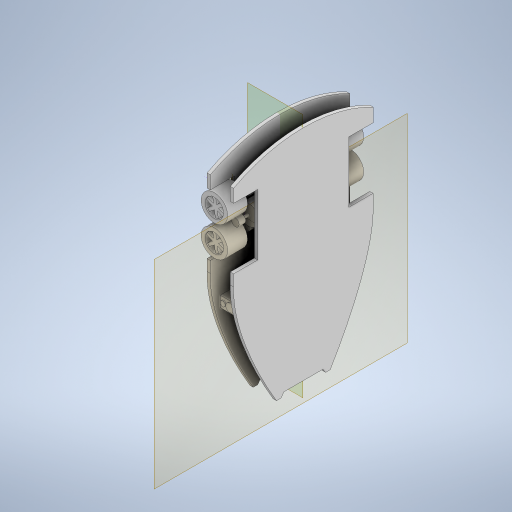
# Autodesk Inventor part: Mickey
Saved by Autodesk Inventor 2024 (Build 280153000, 153)
## iProperties
Created: 2024-01-30
Part Number: Mickey
Material: Generic
Document SubType Name: Modeling
Designer: Hitesh
Density: 1 g/cm^3
Appearance: Default
Author: Hitesh
Autodesk Inventor part; units mm, degrees
ref_plane "YZ Plane" through (0, 0, 0) normal (1, 0, 0) x (0, 1, 0)
ref_plane "XZ Plane" through (0, 0, 0) normal (0, 1, 0) x (-1, 0, 0)
ref_plane "XY Plane" through (0, 0, 0) normal (0, 0, 1) x (1, 0, 0)
sketch "Sketch1" plane through (0, 0, 0) normal (1, 0, 0) x (0, 1, 0)
  line L0 (79.528373, 42.408531) -> (71.671582, 42.408531)
  line L1 (34.839879, 42.408531) -> (28.023668, 42.408531)
  spline S0 degree 3 poles (28.023668, 42.408531) (8.43226, 43.15614) (-20.679837, 30.735066) (-44.361404, 16.548455) knots 0 0 0 0 1 1 1 1
  line L2 (-44.361404, 16.548455) -> (-44.361404, 13.844569)
  line L3 (-44.361404, 13.844569) -> (-41.928778, 12.127215)
  line L4 (-41.928778, 12.127215) -> (-41.928778, 0.037036)
  arc A0 (79.913681, -41.677922) -> (79.528373, 42.408531) centre (0, 0) ccw
  line L5 (79.913681, -41.677922) -> (71.671582, -41.677922)
  line L6 (34.839879, -41.677922) -> (28.023668, -41.677922)
  spline S1 degree 3 poles (28.023668, -41.677922) (8.431166, -42.471764) (-20.687268, -30.025765) (-44.361404, -15.817846) knots 0 0 0 0 1 1 1 1
  line L7 (-44.361404, -15.817846) -> (-44.361404, -13.113961)
  line L8 (-44.361404, -13.113961) -> (-41.928778, -11.396606)
  line L9 (-41.928778, -11.396606) -> (-41.928778, 0.037036)
  line L10 (34.839879, 42.408531) -> (34.839879, 27.893994)
  line L11 (34.839879, 27.893994) -> (71.671582, 27.893994)
  line L12 (71.671582, 27.893994) -> (71.671582, 42.408531)
  line L13 (34.839879, -41.677922) -> (34.839879, -27.163385)
  line L14 (34.839879, -27.163385) -> (71.671582, -27.163385)
  line L15 (71.671582, -27.163385) -> (71.671582, -41.677922)
  point P0 (9.125075, 40.060022)
  point P1 (-16.837429, 30.888781)
  point P2 (9.126574, -39.354229)
  point P3 (-16.837278, -30.181039)
  constraints: 32 end point, 2 parallel, 2 point on circle, 2 point on line, 2 vertical, 1 centre point, 1 coincident, 1 horizontal, 8 other
extrude "Extrusion1" add sketch "Sketch1" along normal blind 2
sketch "Sketch2" plane through (2, 0, 0) normal (1, 0, 0) x (0, 0, -1)
  line L0 (-42.408531, 71.671582) -> (-27.893994, 71.671582) construction
  line L1 (-27.893994, 34.839879) -> (-42.408531, 34.839879) construction
  line L2 (-42.408531, 71.671582) -> (-42.408531, 34.839879) construction
  line L3 (-42.408531, 53.25573) -> (49.70936, 53.25573) construction
  line L4 (-27.893994, 71.671582) -> (-27.893994, 34.839879) construction
  line L5 (41.677922, 34.839879) -> (27.163385, 34.839879) construction
  line L6 (-11.47496, 42.729901) -> (11.47496, 42.729901) construction
  line L7 (11.47496, 42.729901) -> (11.47496, 26.949856) construction
  line L8 (11.47496, 26.949856) -> (-11.47496, 26.949856) construction
  line L9 (-11.47496, 26.949856) -> (-11.47496, 42.729901) construction
  line L10 (-11.47496, 42.729901) -> (11.47496, 26.949856) construction
  line L11 (11.47496, 42.729901) -> (-11.47496, 26.949856) construction
  line L12 (-11.47496, 34.839879) -> (11.47496, 34.839879)
  line L13 (11.47496, 34.839879) -> (11.47496, 19.846275)
  line L14 (11.47496, 19.846275) -> (-11.47496, 19.846275)
  line L15 (-11.47496, 19.846275) -> (-11.47496, 34.839879)
  line L16 (-7.0791, 16.000261) -> (7.117483, 16.000261)
  line L17 (7.117483, 16.000261) -> (7.117483, 4.324761)
  line L18 (7.117483, 4.324761) -> (-7.0791, 4.324761)
  line L19 (-7.0791, 4.324761) -> (-7.0791, 16.000261)
  point P0 (0, 0)
  point P1 (0, 34.839879)
  constraints: 32 end point, 6 parallel, 4 horizontal, 4 midpoint, 3 perpendicular, 1 vertical
extrude "Extrusion2" add sketch "Sketch2" along normal blind 2
sketch "Sketch3" plane through (2, 0, 0) normal (1, 0, 0) x (0, 0, -1)
  line L0 (7.117483, 16.000261) -> (-7.0791, 16.000261) construction
  line L1 (7.117483, 16.000261) -> (7.117483, 4.324761) construction
  line L2 (-7.0791, 16.000261) -> (7.117483, 16.000261) construction
  line L3 (7.117483, 16.000261) -> (7.117483, 4.324761) construction
  line L4 (7.117483, 4.324761) -> (-7.0791, 4.324761) construction
  line L5 (-7.0791, 4.324761) -> (-7.0791, 16.000261) construction
  line L6 (-6.840727, 16.000261) -> (-6.494492, 16.000261)
  line L7 (-6.494492, 16.000261) -> (-6.494492, 17.001112)
  line L8 (-6.494492, 17.001112) -> (-6.840727, 17.001112)
  line L9 (-6.840727, 17.001112) -> (-6.840727, 16.000261)
  line L10 (-5.820727, 16.000261) -> (-5.474492, 16.000261)
  line L11 (-5.474492, 16.000261) -> (-5.474492, 17.001112)
  line L12 (-5.474492, 17.001112) -> (-5.820727, 17.001112)
  line L13 (-5.820727, 17.001112) -> (-5.820727, 16.000261)
  line L14 (-4.800727, 16.000261) -> (-4.454492, 16.000261)
  line L15 (-4.454492, 16.000261) -> (-4.454492, 17.001112)
  line L16 (-4.454492, 17.001112) -> (-4.800727, 17.001112)
  line L17 (-4.800727, 17.001112) -> (-4.800727, 16.000261)
  line L18 (-3.780727, 16.000261) -> (-3.434492, 16.000261)
  line L19 (-3.434492, 16.000261) -> (-3.434492, 17.001112)
  line L20 (-3.434492, 17.001112) -> (-3.780727, 17.001112)
  line L21 (-3.780727, 17.001112) -> (-3.780727, 16.000261)
  line L22 (-2.760727, 16.000261) -> (-2.414492, 16.000261)
  line L23 (-2.414492, 16.000261) -> (-2.414492, 17.001112)
  line L24 (-2.414492, 17.001112) -> (-2.760727, 17.001112)
  line L25 (-2.760727, 17.001112) -> (-2.760727, 16.000261)
  line L26 (-1.740727, 16.000261) -> (-1.394492, 16.000261)
  line L27 (-1.394492, 16.000261) -> (-1.394492, 17.001112)
  line L28 (-1.394492, 17.001112) -> (-1.740727, 17.001112)
  line L29 (-1.740727, 17.001112) -> (-1.740727, 16.000261)
  line L30 (-0.720727, 16.000261) -> (-0.374492, 16.000261)
  line L31 (-0.374492, 16.000261) -> (-0.374492, 17.001112)
  line L32 (-0.374492, 17.001112) -> (-0.720727, 17.001112)
  line L33 (-0.720727, 17.001112) -> (-0.720727, 16.000261)
  line L34 (0.299273, 16.000261) -> (0.645508, 16.000261)
  line L35 (0.645508, 16.000261) -> (0.645508, 17.001112)
  line L36 (0.645508, 17.001112) -> (0.299273, 17.001112)
  line L37 (0.299273, 17.001112) -> (0.299273, 16.000261)
  line L38 (1.319273, 16.000261) -> (1.665508, 16.000261)
  line L39 (1.665508, 16.000261) -> (1.665508, 17.001112)
  line L40 (1.665508, 17.001112) -> (1.319273, 17.001112)
  line L41 (1.319273, 17.001112) -> (1.319273, 16.000261)
  line L42 (2.339273, 16.000261) -> (2.685508, 16.000261)
  line L43 (2.685508, 16.000261) -> (2.685508, 17.001112)
  line L44 (2.685508, 17.001112) -> (2.339273, 17.001112)
  line L45 (2.339273, 17.001112) -> (2.339273, 16.000261)
  line L46 (3.359273, 16.000261) -> (3.705508, 16.000261)
  line L47 (3.705508, 16.000261) -> (3.705508, 17.001112)
  line L48 (3.705508, 17.001112) -> (3.359273, 17.001112)
  line L49 (3.359273, 17.001112) -> (3.359273, 16.000261)
  line L50 (4.379273, 16.000261) -> (4.725508, 16.000261)
  line L51 (4.725508, 16.000261) -> (4.725508, 17.001112)
  line L52 (4.725508, 17.001112) -> (4.379273, 17.001112)
  line L53 (4.379273, 17.001112) -> (4.379273, 16.000261)
  line L54 (5.399273, 16.000261) -> (5.745508, 16.000261)
  line L55 (5.745508, 16.000261) -> (5.745508, 17.001112)
  line L56 (5.745508, 17.001112) -> (5.399273, 17.001112)
  line L57 (5.399273, 17.001112) -> (5.399273, 16.000261)
  line L58 (6.419273, 16.000261) -> (6.765508, 16.000261)
  line L59 (6.765508, 16.000261) -> (6.765508, 17.001112)
  line L60 (6.765508, 17.001112) -> (6.419273, 17.001112)
  line L61 (6.419273, 17.001112) -> (6.419273, 16.000261)
  line L62 (-7.0791, 10.162511) -> (7.117483, 10.162511) construction
  circle A0 centre (0.019192, 10.162511) radius 1.15053 construction
  line L63 (3.81911, 3.323909) -> (3.81911, 4.324761)
  line L64 (3.81911, 4.324761) -> (3.472876, 4.324761)
  line L65 (3.472876, 3.323909) -> (3.81911, 3.323909)
  line L66 (3.472876, 4.324761) -> (3.472876, 3.323909)
  line L67 (2.79911, 3.323909) -> (2.79911, 4.324761)
  line L68 (2.79911, 4.324761) -> (2.452876, 4.324761)
  line L69 (2.452876, 4.324761) -> (2.452876, 3.323909)
  line L70 (1.77911, 3.323909) -> (1.77911, 4.324761)
  line L71 (1.77911, 4.324761) -> (1.432876, 4.324761)
  line L72 (1.432876, 4.324761) -> (1.432876, 3.323909)
  line L73 (1.432876, 3.323909) -> (1.77911, 3.323909)
  line L74 (2.452876, 3.323909) -> (2.79911, 3.323909)
  line L75 (0.75911, 3.323909) -> (0.75911, 4.324761)
  line L76 (0.412876, 3.323909) -> (0.75911, 3.323909)
  line L77 (0.75911, 4.324761) -> (0.412876, 4.324761)
  line L78 (0.412876, 4.324761) -> (0.412876, 3.323909)
  line L79 (-0.26089, 3.323909) -> (-0.26089, 4.324761)
  line L80 (-0.26089, 4.324761) -> (-0.607124, 4.324761)
  line L81 (-0.607124, 3.323909) -> (-0.26089, 3.323909)
  line L82 (-1.28089, 3.323909) -> (-1.28089, 4.324761)
  line L83 (-1.627124, 4.324761) -> (-1.627124, 3.323909)
  line L84 (-1.28089, 4.324761) -> (-1.627124, 4.324761)
  line L85 (-1.627124, 3.323909) -> (-1.28089, 3.323909)
  line L86 (-0.607124, 4.324761) -> (-0.607124, 3.323909)
  line L87 (-2.30089, 3.323909) -> (-2.30089, 4.324761)
  line L88 (-2.647124, 3.323909) -> (-2.30089, 3.323909)
  line L89 (-2.30089, 4.324761) -> (-2.647124, 4.324761)
  line L90 (-2.647124, 4.324761) -> (-2.647124, 3.323909)
  line L91 (-3.32089, 3.323909) -> (-3.32089, 4.324761)
  line L92 (-3.32089, 4.324761) -> (-3.667124, 4.324761)
  line L93 (-3.667124, 3.323909) -> (-3.32089, 3.323909)
  line L94 (-4.34089, 3.323909) -> (-4.34089, 4.324761)
  line L95 (-4.34089, 4.324761) -> (-4.687124, 4.324761)
  line L96 (-4.687124, 3.323909) -> (-4.34089, 3.323909)
  line L97 (-5.36089, 3.323909) -> (-5.36089, 4.324761)
  line L98 (-5.36089, 4.324761) -> (-5.707124, 4.324761)
  line L99 (-5.707124, 3.323909) -> (-5.36089, 3.323909)
  line L100 (-6.38089, 3.323909) -> (-6.38089, 4.324761)
  line L101 (-6.38089, 4.324761) -> (-6.727124, 4.324761)
  line L102 (-6.727124, 4.324761) -> (-6.727124, 3.323909)
  line L103 (-6.727124, 3.323909) -> (-6.38089, 3.323909)
  line L104 (-3.667124, 4.324761) -> (-3.667124, 3.323909)
  line L105 (6.87911, 4.324761) -> (6.532876, 4.324761)
  line L106 (6.532876, 4.324761) -> (6.532876, 3.323909)
  line L107 (6.532876, 3.323909) -> (6.87911, 3.323909)
  line L108 (6.87911, 3.323909) -> (6.87911, 4.324761)
  line L109 (5.85911, 4.324761) -> (5.512876, 4.324761)
  line L110 (5.512876, 4.324761) -> (5.512876, 3.323909)
  line L111 (5.512876, 3.323909) -> (5.85911, 3.323909)
  line L112 (4.492876, 4.324761) -> (4.492876, 3.323909)
  line L113 (4.83911, 4.324761) -> (4.492876, 4.324761)
  line L114 (4.83911, 3.323909) -> (4.83911, 4.324761)
  line L115 (5.85911, 3.323909) -> (5.85911, 4.324761)
  line L116 (4.492876, 3.323909) -> (4.83911, 3.323909)
  line L117 (-4.687124, 4.324761) -> (-4.687124, 3.323909)
  line L118 (-5.707124, 4.324761) -> (-5.707124, 3.323909)
  line L119 (7.117483, 4.324761) -> (-7.0791, 4.324761) construction
  line L120 (8.115724, 15.294592) -> (8.115724, 15.640827)
  line L121 (8.115724, 15.640827) -> (7.117483, 15.640827)
  line L122 (7.117483, 15.640827) -> (7.117483, 15.294592)
  line L123 (7.117483, 15.294592) -> (8.115724, 15.294592)
  line L124 (7.117483, 4.324761) -> (7.117483, 16.000261) construction
  line L125 (7.117483, 14.610827) -> (7.117483, 14.264592)
  line L126 (8.115724, 14.610827) -> (7.117483, 14.610827)
  line L127 (8.115724, 14.264592) -> (8.115724, 14.610827)
  line L128 (7.117483, 14.264592) -> (8.115724, 14.264592)
  line L129 (7.117483, 13.580827) -> (7.117483, 13.234592)
  line L130 (8.115724, 13.580827) -> (7.117483, 13.580827)
  line L131 (8.115724, 13.234592) -> (8.115724, 13.580827)
  line L132 (7.117483, 13.234592) -> (8.115724, 13.234592)
  line L133 (7.117483, 12.550827) -> (7.117483, 12.204592)
  line L134 (8.115724, 12.550827) -> (7.117483, 12.550827)
  line L135 (8.115724, 12.204592) -> (8.115724, 12.550827)
  line L136 (7.117483, 12.204592) -> (8.115724, 12.204592)
  line L137 (7.117483, 11.520827) -> (7.117483, 11.174592)
  line L138 (8.115724, 11.520827) -> (7.117483, 11.520827)
  line L139 (8.115724, 11.174592) -> (8.115724, 11.520827)
  line L140 (7.117483, 11.174592) -> (8.115724, 11.174592)
  line L141 (7.117483, 10.490827) -> (7.117483, 10.144592)
  line L142 (8.115724, 10.490827) -> (7.117483, 10.490827)
  line L143 (8.115724, 10.144592) -> (8.115724, 10.490827)
  line L144 (7.117483, 10.144592) -> (8.115724, 10.144592)
  line L145 (7.117483, 9.460827) -> (7.117483, 9.114592)
  line L146 (8.115724, 9.460827) -> (7.117483, 9.460827)
  line L147 (8.115724, 9.114592) -> (8.115724, 9.460827)
  line L148 (7.117483, 9.114592) -> (8.115724, 9.114592)
  line L149 (7.117483, 8.430827) -> (7.117483, 8.084592)
  line L150 (8.115724, 8.430827) -> (7.117483, 8.430827)
  line L151 (8.115724, 8.084592) -> (8.115724, 8.430827)
  line L152 (7.117483, 8.084592) -> (8.115724, 8.084592)
  line L153 (7.117483, 7.400827) -> (7.117483, 7.054592)
  line L154 (8.115724, 7.400827) -> (7.117483, 7.400827)
  line L155 (8.115724, 7.054592) -> (8.115724, 7.400827)
  line L156 (7.117483, 7.054592) -> (8.115724, 7.054592)
  line L157 (7.117483, 6.370827) -> (7.117483, 6.024592)
  line L158 (8.115724, 6.370827) -> (7.117483, 6.370827)
  line L159 (8.115724, 6.024592) -> (8.115724, 6.370827)
  line L160 (7.117483, 6.024592) -> (8.115724, 6.024592)
  line L161 (7.117483, 5.340827) -> (7.117483, 4.994592)
  line L162 (8.115724, 5.340827) -> (7.117483, 5.340827)
  line L163 (8.115724, 4.994592) -> (8.115724, 5.340827)
  line L164 (7.117483, 4.994592) -> (8.115724, 4.994592)
  line L165 (0.019192, 12.377709) -> (0.019192, 7.657773) construction
  line L166 (-7.0791, 16.000261) -> (-7.0791, 4.324761) construction
  line L167 (-7.0791, 16.000261) -> (-7.0791, 4.324761) construction
  line L168 (-7.0791, 15.294592) -> (-8.077341, 15.294592)
  line L169 (-7.0791, 15.640827) -> (-7.0791, 15.294592)
  line L170 (-8.077341, 15.640827) -> (-7.0791, 15.640827)
  line L171 (-8.077341, 15.294592) -> (-8.077341, 15.640827)
  line L172 (-7.0791, 4.324761) -> (-7.0791, 16.000261) construction
  line L173 (-7.0791, 14.610827) -> (-7.0791, 14.264592)
  line L174 (-8.077341, 14.610827) -> (-7.0791, 14.610827)
  line L175 (-8.077341, 14.264592) -> (-8.077341, 14.610827)
  line L176 (-7.0791, 14.264592) -> (-8.077341, 14.264592)
  line L177 (-7.0791, 13.580827) -> (-7.0791, 13.234592)
  line L178 (-8.077341, 13.580827) -> (-7.0791, 13.580827)
  line L179 (-8.077341, 13.234592) -> (-8.077341, 13.580827)
  line L180 (-7.0791, 13.234592) -> (-8.077341, 13.234592)
  line L181 (-7.0791, 12.550827) -> (-7.0791, 12.204592)
  line L182 (-8.077341, 12.550827) -> (-7.0791, 12.550827)
  line L183 (-8.077341, 12.204592) -> (-8.077341, 12.550827)
  line L184 (-7.0791, 12.204592) -> (-8.077341, 12.204592)
  line L185 (-7.0791, 11.520827) -> (-7.0791, 11.174592)
  line L186 (-8.077341, 11.520827) -> (-7.0791, 11.520827)
  line L187 (-8.077341, 11.174592) -> (-8.077341, 11.520827)
  line L188 (-7.0791, 11.174592) -> (-8.077341, 11.174592)
  line L189 (-7.0791, 10.490827) -> (-7.0791, 10.144592)
  line L190 (-8.077341, 10.490827) -> (-7.0791, 10.490827)
  line L191 (-8.077341, 10.144592) -> (-8.077341, 10.490827)
  line L192 (-7.0791, 10.144592) -> (-8.077341, 10.144592)
  line L193 (-7.0791, 9.460827) -> (-7.0791, 9.114592)
  line L194 (-8.077341, 9.460827) -> (-7.0791, 9.460827)
  line L195 (-8.077341, 9.114592) -> (-8.077341, 9.460827)
  line L196 (-7.0791, 9.114592) -> (-8.077341, 9.114592)
  line L197 (-7.0791, 8.430827) -> (-7.0791, 8.084592)
  line L198 (-8.077341, 8.430827) -> (-7.0791, 8.430827)
  line L199 (-8.077341, 8.084592) -> (-8.077341, 8.430827)
  line L200 (-7.0791, 8.084592) -> (-8.077341, 8.084592)
  line L201 (-7.0791, 7.400827) -> (-7.0791, 7.054592)
  line L202 (-8.077341, 7.400827) -> (-7.0791, 7.400827)
  line L203 (-8.077341, 7.054592) -> (-8.077341, 7.400827)
  line L204 (-7.0791, 7.054592) -> (-8.077341, 7.054592)
  line L205 (-7.0791, 6.370827) -> (-7.0791, 6.024592)
  line L206 (-8.077341, 6.370827) -> (-7.0791, 6.370827)
  line L207 (-8.077341, 6.024592) -> (-8.077341, 6.370827)
  line L208 (-7.0791, 6.024592) -> (-8.077341, 6.024592)
  line L209 (-7.0791, 5.340827) -> (-7.0791, 4.994592)
  line L210 (-8.077341, 5.340827) -> (-7.0791, 5.340827)
  line L211 (-8.077341, 4.994592) -> (-8.077341, 5.340827)
  line L212 (-7.0791, 4.994592) -> (-8.077341, 4.994592)
  point P0 (0, 0)
  dimension "d21" = 1.02
  dimension "d28" = 360
  dimension "d32" = 1.03
  constraints: 420 end point, 48 symmetric about line, 4 parallel, 3 horizontal, 3 midpoint, 2 perpendicular, 2 point on line, 2 vertical, 1 centre point, 1 collinear, 415 other
  measures "d21" distance of L6.start L10.start
  measures "d32" distance of L123.start L125.end
extrude "Extrusion3" add sketch "Sketch3" along normal blind 1.5
sketch "Sketch4" plane through (2, 4.994592, -8.115724) normal (0, -1, 0) x (1, 0, 0)
  line L0 (1.5, 0.998241) -> (0, 0.998241)
  line L1 (0, 0.998241) -> (1, 0.998241)
  line L2 (1, 0.998241) -> (1, 0.498241)
  line L3 (1, 0.498241) -> (0, 0.498241)
  line L4 (0, 0.498241) -> (0, 0.998241)
  line L5 (0, 15.694824) -> (1, 15.694824)
  line L6 (1, 15.694824) -> (1, 15.194824)
  line L7 (1, 15.194824) -> (0, 15.194824)
  line L8 (0, 15.194824) -> (0, 15.694824)
  line L9 (0, 15.194824) -> (2, 15.194824)
  line L10 (0, 20.242939) -> (0, -3.280882)
  point P0 (-2, 8.115724)
  point P1 (1, 0.998241)
  dimension "d39" = 1
  dimension "d40" = 0.5
  dimension "d41" = 1
  dimension "d42" = 0.5
  constraints: 16 end point, 4 parallel, 2 collinear, 2 horizontal, 2 perpendicular
  measures "d39" distance of L2.end L3.end
  measures "d40" distance of L1.end L2.end
  measures "d41" distance of L6.end L7.end
  measures "d42" distance of L5.end L6.end
extrude "Extrusion4" cut sketch "Sketch4" against normal up to surface (14.851683 mm away)
sketch "Sketch5" plane through (2, 16.000261, 6.840727) normal (0, 0, 1) x (1, 0, 0)
  line L0 (0, -11.6755) -> (1, -11.6755)
  line L1 (1, -11.6755) -> (1, -12.1755)
  line L2 (1, -12.1755) -> (0, -12.1755)
  line L3 (0, -12.1755) -> (0, -11.6755)
  line L4 (0, -11.6755) -> (2, -11.6755)
  line L5 (0, -12.676351) -> (0, -11.6755)
  line L6 (0, 0.5) -> (1, 0.5)
  line L7 (1, 0.5) -> (1, 0)
  line L8 (1, 0) -> (0, 0)
  line L9 (0, 0) -> (0, 0.5)
  line L10 (0, 0) -> (2, 0)
  line L11 (0, 0) -> (0, 1.000851)
  point P0 (-2, -16.000261)
  dimension "d45" = 1
  dimension "d46" = 0.5
  dimension "d47" = 1
  dimension "d48" = 0.5
  constraints: 16 end point, 4 collinear, 4 parallel, 2 horizontal, 2 perpendicular
  measures "d45" distance of L1.end L2.end
  measures "d46" distance of L0.end L1.end
  measures "d47" distance of L7.end L8.end
  measures "d48" distance of L6.end L7.end
extrude "Extrusion5" cut sketch "Sketch5" against normal through all
sketch "Sketch6" plane through (0, 34.839879, 27.893994) normal (0, 0, 1) x (1, 0, 0)
  line L0 (0, 36.831703) -> (0, 0) construction
  line L1 (0, 18.415852) -> (14.226225, 18.415852) construction
  line L2 (8.271561, 36.831703) -> (8.271561, 18.415852) construction
  line L3 (8.271561, 27.623777) -> (-16.043318, 27.623777) construction
  line L4 (3.408585, 18.415852) -> (3.408585, 0) construction
  point P0 (0, -34.839879)
  constraints: 8 end point, 2 horizontal, 2 midpoint, 2 point on line, 1 perpendicular, 1 vertical
ref_plane "Work Plane1" through (0, 34.839879, 29.393994) normal (0, 0, 1) x (1, 0, 0)
sketch "Sketch7" plane through (0, 34.839879, 29.393994) normal (0, 0, 1) x (1, 0, 0)
  line L0 (3.388556, 18.455419) -> (3.388556, 36.831703) construction
  circle A0 centre (3.388556, 27.643561) radius 8
  line L1 (3.388556, 18.455419) -> (3.388556, 0.120115) construction
  circle A1 centre (3.388556, 9.287767) radius 8
  point P0 (0, -34.839879)
  dimension "d52" = 16
  dimension "d53" = 16
  constraints: 4 end point, 2 centre point, 2 midpoint, 2 vertical
  measures "d52" diameter of A0
  measures "d53" diameter of A1
extrude "Extrusion6" add sketch "Sketch7" along normal blind 12
sketch "Sketch8" plane through (3.388556, 62.48344, 29.393994) normal (0, 0, -1) x (-1, 0, 0)
  circle A0 centre (0, 0) radius 1.045344 construction
  circle A1 centre (0, 0) radius 0.75
  circle A2 centre (0, -18.355794) radius 8
  circle A3 centre (0, -18.355794) radius 0.75
  point P0 (3.388556, -62.48344)
  dimension "d56" = 1.5
  dimension "d57" = 1.5
  constraints: 3 centre point, 2 coincident
  measures "d56" diameter of A1
  measures "d57" diameter of A3
extrude "Extrusion7" add sketch "Sketch8" along normal blind 6 contours A1 | A3
sketch "Sketch9" plane through (3.388556, 62.48344, 23.393994) normal (0, 0, -1) x (-1, 0, 0)
  circle A0 centre (0, 0) radius 0.75
  arc A1 (1.388556, 2.659307) -> (1.388556, -2.659307) centre (0, 0) ccw
  line L0 (1.388556, 9.188142) -> (1.388556, -27.643561)
  line L1 (1.388556, 2.659307) -> (1.388556, -2.659307)
  circle A2 centre (0, -18.355794) radius 0.75
  arc A3 (1.388556, -15.696487) -> (1.388556, -21.015101) centre (0, -18.355794) ccw
  line L2 (1.388556, -15.696487) -> (1.388556, -21.015101)
  point P0 (3.388556, -62.48344)
  dimension "d60" = 3
  dimension "d61" = 6
  constraints: 4 end point, 4 point on circle, 4 point on line, 2 centre point, 2 coincident
  measures "d60" radius of A1
  measures "d61" diameter of A3
extrude "Extrusion8" add sketch "Sketch9" along normal blind 4 contours A0 | L0 A1 | L0 A3 | A2
sketch "Sketch10" plane through (3.388556, 62.48344, 23.393994) normal (0, 0, 1) x (1, 0, 0)
  line L0 (-1.388556, 9.188142) -> (-1.388556, -27.643561)
  circle A0 centre (4.628085, -9.227709) radius 6.016657
  point P0 (-3.388556, -62.48344)
  constraints: 1 centre point
extrude "Extrusion9" add sketch "Sketch10" along normal blind 2 and the other way blind 16
sketch "Sketch11" plane through (3.388556, 62.48344, 25.393994) normal (0, 0, 1) x (1, 0, 0)
  arc A0 (-1.388556, -9.241554) -> (-1.388556, -9.213864) centre (4.628085, -9.227709) ccw
  circle A1 centre (4.628085, -9.227709) radius 0.75
  point P0 (-3.388556, -62.48344)
  dimension "d69" = 1.5
  constraints: 1 centre point, 1 coincident
  measures "d69" diameter of A1
extrude "Extrusion10" add sketch "Sketch11" along normal blind 8
sketch "Sketch12" plane through (8.016641, 53.25573, 33.393994) normal (0, 0, 1) x (1, 0, 0)
  circle A0 centre (0, 0) radius 2.323265
  circle A1 centre (-4.628085, 9.227709) radius 8
  point P0 (-8.016641, -53.25573)
  constraints: 1 centre point, 1 tangent
extrude "Extrusion11" add sketch "Sketch12" against normal blind 4 contours A0
ref_plane "Work Plane2" through (0, 34.839879, 0.365304) normal (0, 0, -1) x (-1, 0, 0)
mirror "Mirror1" about plane through (0, 34.839879, 0.365304) normal (0, 0, -1) of "Extrusion6", "Extrusion11", "Extrusion10", "Extrusion9", "Extrusion8", "Extrusion7"
sketch "Sketch13" plane through (3.388556, 62.48344, 41.393994) normal (0, 0, 1) x (1, 0, 0)
  circle A0 centre (0, 0) radius 5.585986
  line L0 (-3.794465, -4.201608) -> (4.942451, 2.761097)
  line L1 (4.942451, 2.761097) -> (3.794465, 4.201608)
  line L2 (3.794465, 4.201608) -> (-4.942451, -2.761097)
  line L3 (-4.942451, -2.761097) -> (-3.794465, -4.201608)
  line L4 (-3.794465, -4.201608) -> (3.794465, 4.201608) construction
  line L5 (4.942451, 2.761097) -> (-4.942451, -2.761097) construction
  line L6 (1.741467, -5.386907) -> (0.080046, 5.660837)
  line L7 (-1.741467, 5.386907) -> (-0.080046, -5.660837)
  line L8 (5.535932, -1.185299) -> (-4.862405, 2.89974)
  line L9 (-5.535932, 1.185299) -> (4.862405, -2.89974)
  line L10 (3.794465, 4.201608) -> (-4.942451, -2.761097)
  line L11 (-3.794465, -4.201608) -> (4.942451, 2.761097)
  line L12 (-1.741467, 5.386907) -> (-0.080046, -5.660837)
  line L13 (1.741467, -5.386907) -> (0.080046, 5.660837)
  line L14 (-5.535932, 1.185299) -> (4.862405, -2.89974)
  line L15 (5.535932, -1.185299) -> (-4.862405, 2.89974)
  circle A1 centre (0, -18.330655) radius 5.585986
  line L16 (-3.794465, -22.532263) -> (4.942451, -15.569559)
  line L17 (4.942451, -15.569559) -> (3.794465, -14.129047)
  line L18 (3.794465, -14.129047) -> (-4.942451, -21.091752)
  line L19 (-4.942451, -21.091752) -> (-3.794465, -22.532263)
  line L20 (-3.794465, -22.532263) -> (3.794465, -14.129047) construction
  line L21 (4.942451, -15.569559) -> (-4.942451, -21.091752) construction
  line L22 (1.741467, -23.717562) -> (0.080046, -12.669819)
  line L23 (-1.741467, -12.943748) -> (-0.080046, -23.991492)
  line L24 (5.535932, -19.515954) -> (-4.862405, -15.430915)
  line L25 (-5.535932, -17.145356) -> (4.862405, -21.230395)
  line L26 (3.794465, -14.129047) -> (-4.942451, -21.091752)
  line L27 (-3.794465, -22.532263) -> (4.942451, -15.569559)
  line L28 (-1.741467, -12.943748) -> (-0.080046, -23.991492)
  line L29 (1.741467, -23.717562) -> (0.080046, -12.669819)
  line L30 (-5.535932, -17.145356) -> (4.862405, -21.230395)
  line L31 (5.535932, -19.515954) -> (-4.862405, -15.430915)
  point P0 (-3.388556, -62.48344)
  point P1 (-4.791251, 2.871787)
  point P2 (-1.147986, 1.440512)
  point P3 (-1.730098, 5.311309)
  point P4 (-1.821513, -0.273929)
  point P5 (-5.464777, 1.157346)
  point P6 (-4.882665, -2.713452)
  point P7 (-0.091415, -5.585238)
  point P8 (-0.673527, -1.714441)
  point P9 (-3.734679, -4.153963)
  point P10 (4.791251, -2.871787)
  point P11 (1.147986, -1.440512)
  point P12 (1.730098, -5.311309)
  point P13 (1.821513, 0.273929)
  point P14 (5.464777, -1.157346)
  point P15 (4.882665, 2.713452)
  point P16 (0.091415, 5.585238)
  point P17 (0.673527, 1.714441)
  point P18 (3.734679, 4.153963)
  point P19 (1.147986, -19.771167)
  point P20 (1.730098, -23.641964)
  point P21 (4.791251, -21.202442)
  point P22 (-0.091415, -23.915893)
  point P23 (-0.673527, -20.045096)
  point P24 (-3.734679, -22.484618)
  point P25 (-1.821513, -18.604584)
  point P26 (-5.464777, -17.17331)
  point P27 (-4.882665, -21.044107)
  point P28 (-1.147986, -16.890143)
  point P29 (-1.730098, -13.019346)
  point P30 (-4.791251, -15.458869)
  point P31 (0.091415, -12.745417)
  point P32 (0.673527, -16.616214)
  point P33 (3.734679, -14.176692)
  point P34 (1.821513, -18.056726)
  point P35 (5.464777, -19.488001)
  point P36 (4.882665, -15.617204)
  dimension "d76" = 360
  dimension "d84" = 360
  constraints: 64 end point, 4 midpoint, 4 parallel, 2 centre point, 2 perpendicular, 74 other
extrude "Extrusion12" cut sketch "Sketch13" against normal blind 6 contours A0 L8 L0 | A0 L6 L9 | L2 L6 A0 | A0 L0 L7 | L7 L8 A0 | L2 A0 L9 | A1 L24 L16 | A1 L22 L25 | L18 L22 A1 | A1 L16 L23 | L23 L24 A1 | L18 A1 L25
sketch "Sketch14" plane through (3.388556, 62.48344, 41.393994) normal (0, 0, 1) x (1, 0, 0)
  circle A0 centre (0, 0) radius 5.585986
  arc A1 (1.730098, -23.641964) -> (4.791251, -21.202442) centre (0, -18.330655) ccw
  circle A2 centre (0, -18.330655) radius 5.585986
  point P0 (-3.388556, -62.48344)
  constraints: 2 centre point, 1 coincident
extrude "Extrusion13" cut sketch "Sketch14" against normal blind 0.7
mirror "Mirror2" about plane through (0, 34.839879, 0.365304) normal (0, 0, -1) of "Extrusion13", "Extrusion12", "Extrusion6"
sketch "Sketch15" plane through (2, 0, 0) normal (1, 0, 0) x (0, 0, -1)
  line L0 (-13.844569, -44.361404) -> (-13.844569, 2.739873) construction
  line L1 (-13.844569, 2.739873) -> (13.113961, 2.739873) construction
  line L2 (13.113961, -44.361404) -> (15.817846, -44.361404) construction
  line L3 (13.113961, 2.739873) -> (13.113961, -44.361404) construction
  line L4 (-13.844569, -20.810765) -> (-17.838326, -25.941355)
  line L5 (-17.838326, -25.941355) -> (-22.283823, -22.480889)
  line L6 (-22.283823, -22.480889) -> (-18.290067, -17.350299)
  line L7 (-18.290067, -17.350299) -> (-13.844569, -20.810765)
  line L8 (-30.753552, 13.664836) -> (-30.764664, 7.163074)
  line L9 (-30.764664, 7.163074) -> (-36.39824, 7.172702)
  line L10 (-36.39824, 7.172702) -> (-36.387128, 13.674464)
  line L11 (-36.387128, 13.674464) -> (-30.753552, 13.664836)
  point P0 (0, 0)
  constraints: 22 end point, 4 parallel, 4 perpendicular, 1 midpoint, 1 vertical
extrude "Extrusion14" add sketch "Sketch15" along normal blind 9
sketch "Sketch16" plane through (2, -25.941355, 17.838326) normal (0, -0.7891064, 0.6142566) x (1, 0, 0)
  line L0 (0, 5.633584) -> (9, 5.633584) construction
  line L1 (0, 0) -> (9, 0) construction
  line L2 (0, 5.633584) -> (9, 0) construction
  line L3 (6.271221, -0.889158) -> (6.271221, 3.293106)
  circle A0 centre (6.271221, 2.816792) radius 2.517328
  circle A1 centre (1.994855, 2.816792) radius 1.587953
  point P0 (-2, 1.858311)
  constraints: 2 centre point, 2 end point, 1 point on line
extrude "Extrusion15" add sketch "Sketch16" along normal blind 0.5
sketch "Sketch17" plane through (2, 7.172702, 36.39824) normal (0, 0.001709, 0.9999985) x (1, 0, 0)
  circle A0 centre (6.240376, 3.24716) radius 2.517328
  circle A1 centre (1.964009, 3.24716) radius 1.587953
  line L0 (0, 6.501772) -> (9, 6.501772) construction
  line L1 (4.5, 6.501772) -> (4.5, 0) construction
  line L2 (0, 0) -> (9, 0) construction
  line L3 (0, 6.501772) -> (0, 0) construction
  line L4 (0, 3.250886) -> (9, 3.250886) construction
  line L5 (9, 6.501772) -> (9, 0) construction
  point P0 (-2, -7.110485)
  constraints: 4 end point, 4 midpoint, 2 centre point
extrude "Extrusion16" add sketch "Sketch17" along normal blind 0.5
mirror "Mirror3" about plane through (0, 34.839879, 0.365304) normal (0, 0, -1) of "Extrusion16", "Extrusion14", "Extrusion15"
ref_plane "Work Plane3" through (14.033298, 53.25573, 25.393994) normal (1, 0, 0) x (0, 1, 0)
sketch "Sketch18" plane through (14.033298, 53.25573, 25.393994) normal (1, 0, 0) x (0, 1, 0)
  line L0 (26.272658, 17.014559) -> (18.415867, 17.014559)
  line L1 (-18.415836, 17.014559) -> (-25.232047, 17.014559)
  spline S0 degree 3 poles (-25.232047, 17.014559) (-44.820329, 17.749971) (-73.933178, 5.33616) (-97.617119, -8.845517) knots 0 0 0 0 1 1 1 1
  line L2 (-97.617119, -8.845517) -> (-97.617119, -11.549402)
  line L3 (-97.617119, -11.549402) -> (-95.184493, -13.266757)
  line L4 (-95.184493, -13.266757) -> (-95.184493, -25.356936)
  arc A0 (26.657966, -67.071894) -> (26.272658, 17.014559) centre (-53.255715, -25.393972) ccw
  line L5 (26.657966, -67.071894) -> (18.415867, -67.071894)
  spline S1 degree 3 poles (-25.232047, -67.071894) (-44.82455, -67.865774) (-73.943009, -55.419375) (-97.617119, -41.211818) knots 0 0 0 0 1 1 1 1
  line L6 (-18.415836, -67.071894) -> (-25.232047, -67.071894)
  line L7 (-97.617119, -41.211818) -> (-97.617119, -38.507933)
  line L8 (-97.617119, -38.507933) -> (-95.184493, -36.790578)
  line L9 (-95.184493, -36.790578) -> (-95.184493, -25.356936)
  line L10 (-18.415836, 17.014559) -> (-18.415836, 2.500022)
  line L11 (-18.415836, 2.500022) -> (18.415867, 2.500022)
  line L12 (18.415867, 2.500022) -> (18.415867, 17.014559)
  line L13 (-18.415836, -67.071894) -> (-18.415836, -52.557357)
  line L14 (-18.415836, -52.557357) -> (18.415867, -52.557357)
  line L15 (18.415867, -52.557357) -> (18.415867, -67.071894)
  line L16 (7.319073, 0.244522) -> (-6.993029, 0.244522)
  line L17 (-6.993029, 0.244522) -> (-6.993029, -50.447503)
  line L18 (-6.993029, -50.447503) -> (7.319073, -50.447503)
  line L19 (7.319073, -50.447503) -> (7.319073, 0.244522)
  point P0 (-53.25573, -25.393994)
  point P1 (-44.128344, 14.659963)
  point P2 (-70.091167, 5.489571)
  point P3 (-44.129163, -64.748149)
  point P4 (-70.093073, -55.574831)
  constraints: 40 end point, 4 parallel, 2 horizontal, 2 point on circle, 2 point on line, 2 vertical, 1 centre point, 1 coincident, 1 perpendicular, 8 other
extrude "Extrusion17" add sketch "Sketch18" along normal blind 2 contours A0 L5 L15 L14 L13 L6 S1 L7 L8 L9 L4 L3 L2 S0 L1 L10 L11 L12 L0 | L19 L18 L17 L16
body "Solid1"
